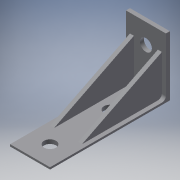
# Autodesk Inventor part: equerre_percage
Saved by Autodesk Inventor 2018.1 (Build 221171000, 171)
## iProperties
Created: 2011-05-02
Part Number: equerre_percage
Material: Aluminum alloy, Wrought
Document SubType Name: Modeling
Designer: Justine
Density: 2 g/cm^3
Mass: 9.85084 g
Surface Area: 53.675 cm^2
Volume: 4.92542 cm^3
Appearance: Default
Author: Justine
Autodesk Inventor part; units mm, degrees
ref_plane "YZ Plane" through (0, 0, 0) normal (1, 0, 0) x (0, 1, 0)
ref_plane "XZ Plane" through (0, 0, 0) normal (0, 1, 0) x (-1, 0, 0)
ref_plane "XY Plane" through (0, 0, 0) normal (0, 0, 1) x (1, 0, 0)
sketch "Sketch1" plane through (0, 0, 0) normal (0, 0, 1) x (1, 0, 0)
  line L0 (-10, 1) -> (10, 1)
  line L1 (10, 1) -> (10, -1)
  line L2 (10, -1) -> (-10, -1)
  line L3 (-10, -1) -> (-10, 1)
  line L4 (-30.9278, 0) -> (36.2543, 0)
  line L5 (0, 23.0241) -> (0, -32.9897)
  point P0 (0, 0)
  dimension "d0" = 20
  dimension "d1" = 2
  constraints: 12 end point, 3 perpendicular, 2 parallel, 2 point on line, 1 horizontal, 2 other
  measures "d0" distance of L0.start L0.end
  measures "d1" distance of L0.end L1.end
sketch "Sketch2" plane through (0, 0, 0) normal (1, 0, 0) x (0, 1, 0)
  line L0 (0, 0) -> (0, -59)
  line L1 (0, -59) -> (30, -59)
  dimension "d2" = 59
  dimension "d3" = 30
  constraints: 4 end point, 1 perpendicular, 1 vertical
  measures "d2" distance of L0.start L0.end
  measures "d3" distance of L0.end L1.end
sweep "Sweep1" add profiles "Sketch1" path "Sketch2"
ref_plane "Work Plane1" through (7, -1, 0) normal (1, 0, 0) x (0, 0, -1)
ref_plane "Work Plane2" through (-7, -1, 0) normal (-1, 0, 0) x (0, 0, 1)
sketch "Sketch3" plane through (7, -1, 0) normal (1, 0, 0) x (0, 0, -1)
  line L0 (58, 22) -> (18, 2)
  line L1 (0, 2) -> (58, 2) projected
  line L2 (58, 2) -> (58, 31) projected
  point P0 (0, 1)
  dimension "d7" = 20
  dimension "d8" = 40
  constraints: 2 end point, 2 point on line
  measures "d7" vertical distance of L0.start L0.end
  measures "d8" horizontal distance of L0.start L0.end
extrude "Rib1" add sketch "Sketch3" along normal mid plane 2 rib yes fills toward (38.0224, 11.9553) open curves L0
sketch "Sketch4" plane through (-7, -1, 0) normal (-1, 0, 0) x (0, 0, 1)
  line L0 (-58, 22) -> (-18, 2)
  line L1 (-58, 2) -> (-58, 31) projected
  line L2 (0, 2) -> (-58, 2) projected
  point P0 (0, 1)
  dimension "d15" = 40
  dimension "d16" = 20
  constraints: 2 end point, 2 point on line
  measures "d15" horizontal distance of L0.start L0.end
  measures "d16" vertical distance of L0.start L0.end
extrude "Rib2" add sketch "Sketch4" along normal mid plane 2 rib yes fills toward (-38.0224, 11.9553) open curves L0
chamfer "Chamfer1" distance 1 angle 45 4 edges at (-10, -1, -30) (0, -1, -60) (10, -1, -30) (0, -1, 0)
fillet "Fillet1" radius 2 3 edges at (0, 1, -58) (-9, 1, -58) (9, 1, -58)
sketch "Sketch5" plane through (-10, 1, 0) normal (0, 1, 0) x (1, 0, 0)
  line L0 (0, 0) -> (20, 0) projected
  line L1 (20, 0) -> (20, 56) projected
  point P0 (10, 0)
  point P1 (10, 10)
  point P2 (10, 40)
  dimension "d27" = 10
  dimension "d28" = 30
  dimension "d29" = 10
  constraints: 1 vertical alignment
  measures "d27" distance from line of L0 point (10, 10)
  measures "d28" distance of point (10, 10) point (10, 40)
  measures "d29" distance from line of L1 point (10, 10)
hole "Hole1" at (0, 1, -10) at (0, 1, -40) direction (0, -1, 0) diameter 6 end through all
sketch "Sketch6" plane through (-10, 30, -58) normal (0, 0, 1) x (1, 0, 0)
  line L0 (20, -27) -> (20, 0) projected
  line L1 (20, 0) -> (0, 0) projected
  point P0 (10, -30)
  point P1 (10, -10)
  dimension "d37" = 10
  dimension "d38" = 10
  measures "d37" distance from line of L1 point (10, -10)
  measures "d38" distance from line of L0 point (10, -10)
hole "Hole2" at (0, 20, -58) direction (0, 0, -1) diameter 6 end through all
body "Solid1"
